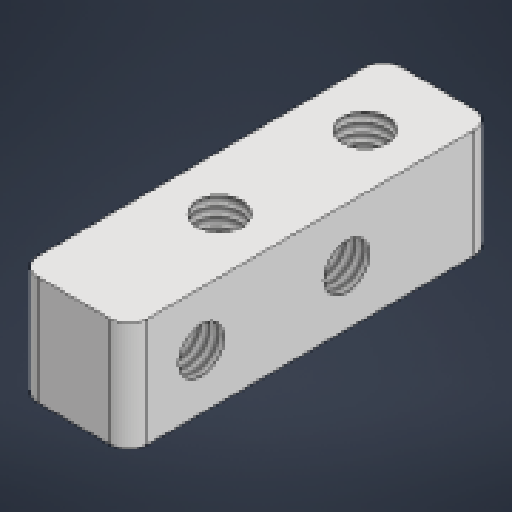
# Autodesk Inventor part: PLATE,NUTBLOCK
Saved by Autodesk Inventor 2026.1 (Build 301233020, 233B)
## iProperties
Created: 2026-01-28
Part Number: PLATE,NUTBLOCK
Material: Aluminum 6061
Document SubType Name: Sheet Metal
Designer: Owen L
Density: 2.7 g/cm^3
Sheet Metal Rule: Default
Appearance: Aluminum - Flat
Author: Owen L
Autodesk Inventor part; units mm, degrees
ref_plane "YZ Plane" through (0, 0, 0) normal (1, 0, 0) x (0, 1, 0)
ref_plane "XZ Plane" through (0, 0, 0) normal (0, 1, 0) x (-1, 0, 0)
ref_plane "XY Plane" through (0, 0, 0) normal (0, 0, 1) x (1, 0, 0)
sketch "Sketch1" plane through (0, 0, 0) normal (0, 1, 0) x (-1, 0, 0)
  line L0 (6.35, 15.875) -> (-6.35, 15.875)
  line L1 (-6.35, 15.875) -> (-6.35, -15.875)
  line L2 (-6.35, -15.875) -> (6.35, -15.875)
  line L3 (6.35, -15.875) -> (6.35, 15.875)
  line L4 (6.35, 15.875) -> (-6.35, -15.875) construction
  line L5 (-6.35, 15.875) -> (6.35, -15.875) construction
  point P0 (0, 0)
  dimension "d0" = 31.75
  dimension "d1" = 12.7
  measures "d0" distance of L0.end L1.end
  measures "d1" distance of L1.end L2.end
extrude "Plate1" add sketch "Sketch1" along normal blind 12.7
sketch "Sketch2" plane through (6.35, 0, 15.875) normal (1, 0, 0) x (0, 0, -1)
  line L0 (0, 0) -> (0, 12.7) construction
  point P0 (15.875, 0)
  point P1 (6.35, 6.35)
  point P2 (19.05, 6.35)
  point P3 (0, 6.35)
  dimension "d3" = 12.7
  dimension "d4" = 6.35
  constraints: 2 horizontal alignment, 1 midpoint
  measures "d3" distance of point (19.05, 6.35) point (6.35, 6.35)
  measures "d4" distance from line of L0 point (6.35, 6.35)
hole "Hole1" at (6.35, 6.35, 9.525) at (6.35, 6.35, -3.175) direction (-1, 0, 0) diameter 3.9624 end through all thread size "10-32 UNF" class "2B" standard "ANSI Unified Screw Threads"
sketch "Sketch3" plane through (0, 12.7, 0) normal (0, 1, 0) x (1, 0, 0)
  point P0 (0, 0)
  point P1 (0, -3.175)
  point P2 (0, 9.525)
  dimension "d12" = 12.7
  dimension "d13" = 3.175
  constraints: 2 vertical alignment
  measures "d12" distance of point (0, 9.525) point (0, -3.175)
  measures "d13" distance of point (0, -3.175) point (0, 0)
hole "Hole2" at (0, 12.7, 3.175) at (0, 12.7, -9.525) direction (0, -1, 0) diameter 3.9624 end through all thread size "10-32 UNF" class "2B" standard "ANSI Unified Screw Threads"
fillet "Corner Round1" radius 1.5875 4 edges at (6.35, 6.35, 15.875) (-6.35, 6.35, 15.875) (-6.35, 6.35, -15.875) (6.35, 6.35, -15.875)
equation "\"d2\" = Thickness"
equation "\"BendRadius\" = Thickness"
equation "\"BendReliefWidth\" = Thickness"
equation "\"BendReliefDepth\" = 0.5 * Thickness"
equation "\"CornerReliefSize\" = 4 * Thickness"
equation "\"MinimumRemnant\" = 2 * Thickness"
equation "\"TransitionRadius\" = BendRadius"
equation "\"JacobiRadiusSize\" = BendRadius"
equation "\"GapSize\" = Thickness"
equation "\"Thickness\" = 12.7"
body "Solid1"
